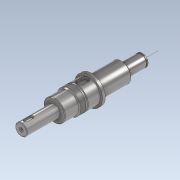
# Autodesk Inventor part: Welle_Passfedernut
Saved by Autodesk Inventor 2022 (Build 260153000, 153)
## iProperties
Created: 2022-03-11
Part Number: Welle_Passfedernut
Material: Edelstahl
Document SubType Name: Modeling
Designer: 123St
Density: 8 g/cm^3
Appearance: Halbpoliert
Mass: 1571.23 g
Surface Area: 267.332 cm^2
Volume: 196.403 cm^3
Shaft_CapstonPart_Dia: 20,000 mm
Passfeder_height: 8,000 mm
Passfeder_width: 12,000 mm
Sprengring_NutBreite: 1,300 mm
Sprengring_NutDurchmesser: 19,000 mm
Flansch_Max_Connector_Lenght: 25,000 mm
Wellennuttiefe_20: 3,500 mm
Nabennuttiefe_20: 2,800 mm
Author: 123St
Autodesk Inventor part; units mm, degrees
ref_plane "YZ Plane" through (0, 0, 0) normal (1, 0, 0) x (0, 1, 0)
ref_plane "XY Plane" through (0, 0, 0) normal (0, 0, 1) x (1, 0, 0)
sketch "Skizze1" plane through (0, 0, 0) normal (1, 0, 0) x (0, 1, 0)
  line L0 (0, 154.8) -> (9, 154.8)
  line L1 (9, 154.8) -> (10, 153.8)
  line L2 (10, 153.8) -> (10, 98.9)
  line L3 (18, 75.9) -> (20, 73.9)
  line L4 (20, 73.9) -> (20, 65.3)
  line L5 (20, 61.3) -> (20, 41.1)
  line L6 (20, 41.1) -> (23.5, 41.1)
  line L7 (23.5, 41.1) -> (23.5, 36.1)
  line L8 (23.5, 36.1) -> (16.5, 36.1)
  line L9 (16.5, 36.1) -> (16.5, -13.8)
  line L10 (10, -15.8) -> (10, -46.7)
  line L11 (10, -46.7) -> (9.5, -46.7)
  line L12 (9.5, -46.7) -> (9.5, -48)
  line L13 (9.5, -48) -> (10, -48)
  line L14 (10, -48) -> (10, -49.5)
  line L15 (10, -49.5) -> (9.5, -50)
  line L16 (9.5, -50) -> (0, -50)
  line L17 (0, -50) -> (0, 154.8)
  line L18 (14.5, -15.8) -> (10, -15.8)
  line L19 (16.5, -13.8) -> (14.5, -15.8)
  line L20 (0, 195.76) -> (0, -90.96) construction
  line L21 (-4.7, 0) -> (28.2, 0) construction
  line L22 (10, 98.9) -> (0, 98.9) construction
  line L23 (10, -15.8) -> (0, -15.8) construction
  line L24 (10, -46.7) -> (0, -46.7) construction
  line L25 (17, 98.9) -> (10, 98.9)
  line L26 (18, 75.9) -> (18, 97.9)
  line L27 (18, 97.9) -> (17, 98.9)
  line L28 (10, 129.8) -> (0, 129.8) construction
  circle A0 centre (20, 63.3) radius 2 construction
  line L29 (20, 65.3) -> (19.0799, 64.3799)
  line L30 (19.0799, 64.3799) -> (19.0799, 62.2201)
  line L31 (19.0799, 62.2201) -> (20, 61.3)
  line L32 (20, 63.3) -> (19.0799, 63.3) construction
  point P0 (0, 0)
  point P1 (18, 98.9)
  dimension "d4" = 45
  dimension "d6" = 1.3
  dimension "d9" = 23.5
  dimension "d11" = 5
  dimension "d19" = 45
  dimension "d20" = 2
  dimension "d21" = 2
  dimension "d22" = 1
  dimension "d34" = 0
  dimension "d35" = 50
  dimension "d36" = 45
  dimension "d87" = 114.7
  dimension "d88" = 0
  dimension "d89" = 30.9
  dimension "d90" = 19
  dimension "d91" = 20
  dimension "d119" = 20
  dimension "d120" = 1.5
  dimension "d122" = 1
  dimension "d123" = 1
  dimension "d124" = 33
  dimension "d125" = 40
  dimension "d126" = 30.9
  dimension "d127" = 25
  dimension "d135" = 78.9
  dimension "d139" = 91.5
  dimension "d140" = 113.7
  dimension "d141" = 22.2
  dimension "d142" = 45
  dimension "d143" = 45
  dimension "d144" = 38.1598
  dimension "d145" = 8.6
  constraints: 62 end point, 13 perpendicular, 12 point on line, 4 vertical, 2 parallel, 2 point on circle, 1 centre point, 1 collinear, 1 horizontal, 1 midpoint
  measures "d4" angle of L17 L15
  measures "d6" distance between parallel lines of L13 L11
  measures "d9" distance from line of L17 L7.end
  measures "d11" distance between parallel lines of L8 L6
  measures "d19" angle of L17 L1
  measures "d20" horizontal distance of L3.start L3.end
  measures "d21" horizontal distance of L18.start L9.end
  measures "d22" horizontal distance of L0.end L1.end
  measures "d34" distance between parallel lines of L20 L17
  measures "d35" distance between parallel lines of L21 L16
  measures "d36" angle of L17 L19
  measures "d87" distance between parallel lines of L22 L23
  measures "d88" distance between parallel lines of L24 L11
  measures "d89" distance between parallel lines of L24 L23
  measures "d90" diameter of L12 L20
  measures "d91" diameter of L10 L20
  measures "d119" diameter of L2 L20
  measures "d120" distance from line of L13 L14.end
  measures "d122" distance of L26.end point (18, 98.9)
  measures "d123" distance of L25.start point (18, 98.9)
  measures "d124" diameter of L9 L17
  measures "d125" diameter of L5 L20
  measures "d126" distance between parallel lines of L22 L28
  measures "d127" distance between parallel lines of L0 L28
  measures "d135" distance from line of L0 L3.start
  measures "d139" distance from line of L0 L32.start
  measures "d140" distance between parallel lines of L6 L0
  measures "d141" distance from line of L6 L32.start
  measures "d142" angle of L30 L29
  measures "d143" angle of L30 L31
  measures "d144" diameter of L30 L17
  measures "d145" distance of L4.end L3.end
revolve "Umdrehung1" add sketch "Skizze1" angle 360 about axis through (0, 0, -50) along (0, 0, 1)
ref_plane "Wellennuttiefe_Arbeitsebene" through (0, 15, 51.2) normal (0, 1, 0) x (-1, 0, 0)
ref_plane "Arbeitsebene1" through (0, 20, 51.2) normal (0, 1, 0) x (-1, 0, 0)
sketch "Skizze2" plane through (0, 20, 51.2) normal (0, 1, 0) x (-1, 0, 0)
  line L0 (0, 9.9) -> (0, -10.1) construction
  line L1 (6, 3.9) -> (6, -4.1)
  line L2 (-6, -4.1) -> (-6, 3.9)
  arc A0 (6, 3.9) -> (-6, 3.9) centre (0, 3.9) ccw
  arc A1 (-6, -4.1) -> (6, -4.1) centre (0, -4.1) ccw
  line L3 (-23.5, -10.1) -> (23.5, -10.1) construction
  line L4 (0, 144.56) -> (0, -142.16) construction
  point P0 (0, -51.2)
  point P1 (0, -0.1)
  dimension "d29" = 20
  dimension "d30" = 12
  constraints: 8 end point, 6 point on circle, 5 tangent, 2 centre point, 2 point on line, 1 collinear, 1 midpoint, 1 parallel, 1 vertical
  measures "d29" distance of L0.start L0.end
  measures "d30" distance between parallel lines of L2 L1
extrude "Passfeder_Ausnahme" cut sketch "Skizze2" against normal up to surface (5 mm away)
thread "Gewinde1" size "M40x1.5" class "6g" standard "ISO Metric profile" full length
ref_plane "Arbeitsebene5" through (0, 10, 126.35) normal (0, 1, 0) x (-1, 0, 0)
sketch "Skizze7" plane through (0, 10, 126.35) normal (0, 1, 0) x (-1, 0, 0)
  line L0 (-10, -27.45) -> (10, -27.45) construction
  line L1 (10, 3.45) -> (-10, 3.45) construction
  line L2 (-10, -27.45) -> (10, -27.45) construction
  line L3 (0, -27.45) -> (0, 3.45) construction
  line L4 (10, 27.45) -> (10, -27.45) construction
  line L5 (-10, 27.45) -> (-10, -27.45) construction
  line L6 (0, 10.95) -> (0, 20.95) construction
  line L7 (3, 10.95) -> (3, 20.95)
  line L8 (-3, 20.95) -> (-3, 10.95)
  arc A0 (-3, 10.95) -> (3, 10.95) centre (0, 10.95) ccw
  arc A1 (3, 20.95) -> (-3, 20.95) centre (0, 20.95) ccw
  line L9 (0, 7.95) -> (3, 7.95) construction
  line L10 (-9, 28.45) -> (9, 28.45) construction
  line L11 (-17, -27.45) -> (17, -27.45) construction
  line L12 (0, 28.45) -> (0, 3.45) construction
  point P0 (0, -126.35)
  point P1 (0, 15.95)
  point P2 (0, 23.95)
  dimension "d100" = 30.9
  dimension "d101" = 6
  dimension "d102" = 16
  dimension "Flansch_Max_Connector_Lenght" = 25
  constraints: 18 end point, 6 point on circle, 5 midpoint, 5 tangent, 4 point on line, 2 centre point, 2 collinear, 2 horizontal, 2 vertical, 1 parallel, 1 perpendicular
  measures "d100" distance between parallel lines of L2 L1
  measures "d101" distance between parallel lines of L8 L7
  measures "d102" distance of L9.start point (0, 23.95)
  measures "Flansch_Max_Connector_Lenght" distance between parallel lines of L1 L10
ref_plane "Wellennuttiefe_Arbeitsebene_2" through (0, 6.5, 126.35) normal (0, 1, 0) x (-1, 0, 0)
extrude "PassfederNut_HeadSide" cut sketch "Skizze7" against normal up to surface (3.5 mm away)
sketch "Skizze9" plane through (0, 0, 154.8) normal (0, 0, 1) x (1, 0, 0)
  circle A0 centre (0, 0) radius 9 construction
  point P0 (0, 0)
  constraints: 1 coincident
hole "Bohrung1" at (0, 0, 154.8) direction (0, 0, -1) diameter 4.134 depth 15 tip angle 118 thread size "M5x0.8" class "6H" standard "ISO Metric profile"
chamfer "Fase4" distance 1.5 angle 45 1 edges at (0, 2.067, 154.8)
equation "\"d6\" = Sprengring_NutBreite"
equation "\"d87\" = -MainAxis_Bearing_Fix2ScrewLimit_Dist + Gestell_Lager_Distanz - MainAxis_Bearing_Fix2Limit_Dist"
equation "\"d89\" = MainAxis_Bearing_Fix2Limit_Dist + MainAxis_Bearing_Fix2ScrewLimit_Dist"
equation "\"d90\" = Sprengring_NutDurchmesser"
equation "\"d91\" = P204_ShaftDiameter"
equation "\"d119\" = P204_ShaftDiameter"
equation "\"d29\" = Passfeder_length"
equation "\"d100\" = MainAxis_Bearing_Fix2ScrewLimit_Dist + MainAxis_Bearing_Fix2Limit_Dist"
equation "\"Wellennuttiefe_20\" = 3.5"
equation "\"Nabennuttiefe_20\" = 2.8"
equation "\"Sprengring_NutBreite\" = 1.3"
equation "\"Sprengring_NutDurchmesser\" = 19"
equation "\"Nabennuttiefe_40\" = 3.3"
equation "\"Wellennuttiefe_40\" = 5"
equation "\"Passfeder_Width_20\" = 6"
equation "\"Passfeder_Width_40\" = 12"
equation "\"MainAxis_Bearing_Fix2ScrewLimit_Dist\" = 23.4"
equation "\"Gestell_Lager_Distanz\" = 145.6"
equation "\"MainAxis_Bearing_Fix2Limit_Dist\" = 7.5"
equation "\"P204_ShaftDiameter\" = 20"
equation "\"Passfeder_length\" = 20"
